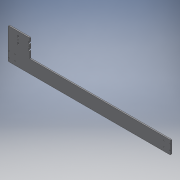
# Autodesk Inventor part: Wiper_Arm_1
Saved by Autodesk Inventor 2019 (Build 230136000, 136)
## iProperties
Created: 2020-03-11
Part Number: Wiper_Arm_1
Material: Generic
Document SubType Name: Modeling
Designer: Vijay
Density: 1 g/cm^3
Appearance: Default
Author: Vijay
Autodesk Inventor part; units mm, degrees
ref_plane "YZ Plane" through (0, 0, 0) normal (1, 0, 0) x (0, 1, 0)
ref_plane "XZ Plane" through (0, 0, 0) normal (0, 1, 0) x (-1, 0, 0)
ref_plane "XY Plane" through (0, 0, 0) normal (0, 0, 1) x (1, 0, 0)
sketch "Sketch1" plane through (0, 0, 0) normal (0, 0, 1) x (1, 0, 0)
  line L0 (19.3072, -32.4) -> (25.8072, -32.4) construction
  line L1 (25.8072, 0) -> (25.8072, -32.4) construction
  line L2 (19.3072, 0) -> (25.8072, 0) construction
  line L3 (19.3072, 0) -> (19.3072, -32.4) construction
  circle A0 centre (22.9072, -6.2) radius 1.75 construction
  circle A1 centre (22.9072, -26.2) radius 1.75 construction
  line L4 (0.0072, -32.4) -> (6.5072, -32.4) construction
  line L5 (6.5072, 0) -> (6.5072, -32.4) construction
  line L6 (0, 0) -> (6.5072, 0) construction
  line L7 (0.0072, 0) -> (0.0072, -32.4) projected
  circle A2 centre (2.9072, -6.2) radius 1.75 construction
  circle A3 centre (2.9072, -26.2) radius 1.75 construction
  line L8 (560.3075, -32.4001) -> (566.8075, -32.4001) construction
  line L9 (566.8075, -0.0001) -> (566.8075, -32.4001) projected
  line L10 (560.3075, -0.0001) -> (566.8075, -0.0001) construction
  line L11 (560.3075, -0.0001) -> (560.3075, -32.4001) construction
  circle A4 centre (563.9075, -6.2001) radius 1.75 construction
  circle A5 centre (563.9075, -26.2001) radius 1.75 construction
  line L12 (541.0075, -32.4001) -> (547.5075, -32.4001) construction
  line L13 (547.5075, -0.0001) -> (547.5075, -32.4001) construction
  line L14 (541.0075, -0.0001) -> (547.5075, -0.0001) construction
  line L15 (541.0075, -0.0001) -> (541.0075, -32.4001) construction
  circle A6 centre (543.9075, -6.2001) radius 1.75 construction
  circle A7 centre (543.9075, -26.2001) radius 1.75 construction
  line L16 (541.9075, 6.4999) -> (565.9075, 6.4999) projected
  line L17 (565.9075, -38.9001) -> (541.9075, -38.9001) projected
  line L18 (566.7649, -38.9) -> (0, -38.9)
  line L19 (0, -38.9) -> (0, 6.5)
  line L20 (0, 6.5) -> (566.7649, 6.5)
  line L21 (566.7649, 6.5) -> (566.7649, -38.9)
  circle A8 centre (563.9075, -26.2001) radius 1.5
  circle A9 centre (563.9075, -6.2001) radius 1.5
  circle A10 centre (543.9075, -26.2001) radius 1.5
  circle A11 centre (543.9075, -6.2001) radius 1.5
  circle A12 centre (22.9072, -26.2) radius 1.5
  circle A13 centre (22.9072, -6.2) radius 1.5
  circle A14 centre (2.9072, -26.2) radius 1.5
  circle A15 centre (2.9072, -6.2) radius 1.5
  point P0 (0, 0)
  dimension "d0" = 3
  dimension "d1" = 3
  dimension "d2" = 3
  dimension "d3" = 3
  dimension "d4" = 3
  dimension "d5" = 3
  dimension "d6" = 3
  dimension "d7" = 3
  constraints: 8 centre point, 8 coincident, 8 end point, 2 parallel, 1 horizontal, 1 perpendicular, 2 other
  measures "d0" diameter of A8
  measures "d1" diameter of A9
  measures "d2" diameter of A10
  measures "d3" diameter of A11
  measures "d4" diameter of A12
  measures "d5" diameter of A13
  measures "d6" diameter of A14
  measures "d7" diameter of A15
extrude "Extrusion1" add sketch "Sketch1" along normal blind 4
fillet "Fillet1" radius 2 4 edges at (566.7649, 6.5, 2) (566.7649, -38.9, 2) (0, -38.9, 2) (0, 6.5, 2)
sketch "Sketch2" plane through (0, 0, 4) normal (0, 0, 1) x (1, 0, 0)
  arc A0 (2, 6.5) -> (0, 4.5) centre (2, 4.5) ccw projected
  line L0 (0, 4.5) -> (0, -36.9) projected
  arc A1 (0, -36.9) -> (2, -38.9) centre (2, -36.9) ccw projected
  line L1 (2, -38.9) -> (564.7649, -38.9) projected
  arc A2 (564.7649, -38.9) -> (566.7649, -36.9) centre (564.7649, -36.9) ccw projected
  line L2 (566.7649, -36.9) -> (566.7649, 4.5) projected
  arc A3 (566.7649, 4.5) -> (564.7649, 6.5) centre (564.7649, 4.5) ccw projected
  line L3 (564.7649, 6.5) -> (2, 6.5) projected
  line L4 (0, 4.5) -> (0, -36.9) projected
  line L5 (0, 4.5) -> (74.776, 4.5)
  line L6 (74.776, 4.5) -> (74.776, 69.6091)
  line L7 (74.776, 69.6091) -> (0, 69.6091)
  line L8 (0, 69.6091) -> (0, 4.5)
  point P0 (0, 0)
  constraints: 8 end point, 2 parallel, 1 horizontal, 1 perpendicular
extrude "Extrusion2" add sketch "Sketch2" against normal up to surface (4 mm away) contours L3 L6 L5 A0 | A0 L8 L7 L6 L3
fillet "Fillet2" radius 2 2 edges at (0, 69.6091, 2) (74.776, 69.6091, 2)
fillet "Fillet3" radius 2 1 edges at (74.776, 6.5, 2)
sketch "Sketch3" plane through (0, 0, 0) normal (0, 0, -1) x (-1, 0, 0)
  line L0 (-32.9952, 56.8458) -> (-32.9952, 50.8458) construction
  line L1 (-32.9952, 56.8458) -> (-36.9952, 56.8458) construction
  line L2 (-36.9952, 50.8458) -> (-36.9952, 56.8458) construction
  line L3 (-32.9952, 50.8458) -> (-36.9952, 50.8458) construction
  line L4 (-32.9952, 35.6458) -> (-32.9952, 29.6458) construction
  line L5 (-32.9952, 35.6458) -> (-36.9952, 35.6458) construction
  line L6 (-36.9952, 29.6458) -> (-36.9952, 35.6458) construction
  line L7 (-32.9952, 29.6458) -> (-36.9952, 29.6458) construction
  line L8 (-70.776, 35.6458) -> (-70.776, 29.6458) construction
  line L9 (-70.776, 35.6458) -> (-74.776, 35.6458) construction
  line L10 (-74.776, 29.6458) -> (-74.776, 35.6458) construction
  line L11 (-70.776, 29.6458) -> (-74.776, 29.6458) construction
  line L12 (-70.776, 56.8458) -> (-70.776, 50.8458) construction
  line L13 (-70.776, 56.8458) -> (-74.776, 56.8458) construction
  line L14 (-74.776, 50.8458) -> (-74.776, 56.8458) construction
  line L15 (-70.776, 50.8458) -> (-74.776, 50.8458) construction
  line L16 (-36.9951, 41.5458) -> (-36.9951, 44.9458) construction
  line L17 (-32.9951, 41.5458) -> (-36.9951, 41.5458) construction
  line L18 (-32.9951, 44.9458) -> (-32.9951, 41.5458) construction
  line L19 (-32.9951, 44.9458) -> (-36.9951, 44.9458) construction
  line L20 (-74.776, 41.5458) -> (-74.776, 44.9458) construction
  line L21 (-70.776, 41.5458) -> (-74.776, 41.5458) construction
  line L22 (-70.776, 44.9458) -> (-70.776, 41.5458) construction
  line L23 (-70.776, 44.9458) -> (-74.776, 44.9458) construction
  line L24 (-74.976, 57.0458) -> (-70.576, 57.0458)
  line L25 (-70.576, 57.0458) -> (-70.576, 50.6458)
  line L26 (-70.576, 50.6458) -> (-74.976, 50.6458)
  line L27 (-74.976, 50.6458) -> (-74.976, 57.0458)
  line L28 (-74.976, 35.8458) -> (-70.576, 35.8458)
  line L29 (-70.576, 35.8458) -> (-70.576, 29.4458)
  line L30 (-70.576, 29.4458) -> (-74.976, 29.4458)
  line L31 (-74.976, 29.4458) -> (-74.976, 35.8458)
  line L32 (-37.1952, 57.0458) -> (-32.7952, 57.0458)
  line L33 (-32.7952, 57.0458) -> (-32.7952, 50.6458)
  line L34 (-32.7952, 50.6458) -> (-37.1952, 50.6458)
  line L35 (-37.1952, 50.6458) -> (-37.1952, 57.0458)
  line L36 (-37.1952, 35.8458) -> (-32.7952, 35.8458)
  line L37 (-32.7952, 35.8458) -> (-32.7952, 29.4458)
  line L38 (-32.7952, 29.4458) -> (-37.1952, 29.4458)
  line L39 (-37.1952, 29.4458) -> (-37.1952, 35.8458)
  circle A0 centre (-72.776, 43.2458) radius 1.6
  circle A1 centre (-34.988, 43.2458) radius 1.6
  point P0 (0, 0)
  dimension "d15" = 0.2
  dimension "d16" = 0.2
  dimension "d17" = 0.2
  dimension "d18" = 0.2
  dimension "d19" = 3.2
  dimension "d20" = 3.2
  constraints: 32 end point, 2 centre point, 12 other
  measures "d15" distance between parallel lines of L13 L24
  measures "d16" distance between parallel lines of L9 L28
  measures "d17" distance between parallel lines of L1 L32
  measures "d18" distance between parallel lines of L5 L36
  measures "d19" diameter of A0
  measures "d20" diameter of A1
extrude "Extrusion3" cut sketch "Sketch3" against normal blind 25.4
sketch "Sketch6" plane through (0, 0, 4) normal (0, 0, 1) x (1, 0, 0)
  line L0 (2, -38.9) -> (564.7649, -38.9) construction
  line L1 (282.6988, 626.8336) -> (282.6988, -296.2495) construction
  line L2 (497.6988, -38.9) -> (67.6988, -38.9)
  line L3 (67.6988, -38.9) -> (67.6988, -34.4)
  line L4 (67.6988, -34.4) -> (497.6988, -34.4)
  line L5 (497.6988, -34.4) -> (497.6988, -38.9)
  point P0 (0, 0)
  dimension "d29" = 4.5
  dimension "d30" = 430
  constraints: 10 end point, 2 parallel, 1 horizontal, 1 perpendicular, 1 point on line, 1 vertical, 1 other
  measures "d29" distance of L4.end L2.start
  measures "d30" distance of L3.end L4.end
extrude "Extrusion5" cut sketch "Sketch6" against normal blind 25.4
fillet "Fillet5" radius 1 2 edges at (497.6988, -38.9, 2) (67.6988, -38.9, 2)
sketch "Sketch7" plane through (0, 0, 4) normal (0, 0, 1) x (1, 0, 0)
  arc A0 (214.4105, 1.0634) -> (213.9105, 1.5634) centre (213.9105, 1.0634) ccw construction
  line L0 (213.9105, 1.5634) -> (210.4105, 1.5634) construction
  line L1 (210.4105, 1.5634) -> (210.4105, 8.4392) construction
  line L2 (210.4105, 8.4392) -> (201.1321, 8.4392) construction
  arc A1 (201.1321, 8.4392) -> (199.8552, 7.9785) centre (201.1321, 6.4392) ccw construction
  line L3 (199.8552, 7.9785) -> (161.5461, -23.8002) construction
  arc A2 (161.5461, -23.8002) -> (160.823, -25.3395) centre (162.823, -25.3395) ccw construction
  line L4 (160.823, -25.3395) -> (160.823, -34.4) projected
  line L5 (160.823, -34.4) -> (167.6988, -34.4) projected
  line L6 (167.6988, -34.4) -> (167.6988, -37.9) projected
  arc A3 (167.6988, -37.9) -> (168.1988, -38.4) centre (168.1988, -37.9) ccw projected
  line L7 (168.1988, -38.4) -> (173.1988, -38.4) projected
  arc A4 (173.1988, -38.4) -> (173.6988, -37.9) centre (173.1988, -37.9) ccw projected
  line L8 (173.6988, -37.9) -> (173.6988, -34.4) projected
  line L9 (173.6988, -34.4) -> (179.5988, -34.4) projected
  line L10 (179.5988, -34.4) -> (179.5988, -28.6) projected
  line L11 (179.5988, -28.6) -> (178.3488, -28.6) construction
  line L12 (178.3488, -28.6) -> (178.3488, -26.2) construction
  line L13 (178.3488, -26.2) -> (179.5988, -26.2) construction
  line L14 (179.5988, -26.2) -> (179.5988, -23.55) construction
  line L15 (179.5988, -23.55) -> (182.9988, -23.55) construction
  line L16 (182.9988, -23.55) -> (182.9988, -26.2) construction
  line L17 (182.9988, -26.2) -> (184.2488, -26.2) construction
  line L18 (184.2488, -26.2) -> (184.2488, -28.6) construction
  line L19 (184.2488, -28.6) -> (182.9988, -28.6) construction
  line L20 (182.9988, -28.6) -> (182.9988, -34.4) projected
  line L21 (182.9988, -34.4) -> (188.8988, -34.4) projected
  line L22 (188.8988, -34.4) -> (188.8988, -37.9) projected
  arc A5 (188.8988, -37.9) -> (189.3988, -38.4) centre (189.3988, -37.9) ccw projected
  line L23 (189.3988, -38.4) -> (194.3988, -38.4) projected
  arc A6 (194.3988, -38.4) -> (194.8988, -37.9) centre (194.3988, -37.9) ccw projected
  line L24 (194.8988, -37.9) -> (194.8988, -34.4) projected
  line L25 (194.8988, -34.4) -> (210.4105, -34.4) projected
  line L26 (210.4105, -34.4) -> (210.4105, -25.6366) projected
  line L27 (210.4105, -25.6366) -> (213.9105, -25.6366) construction
  arc A7 (213.9105, -25.6366) -> (214.4105, -25.1366) centre (213.9105, -25.1366) ccw construction
  line L28 (214.4105, -25.1366) -> (214.4105, -20.1366) construction
  arc A8 (214.4105, -20.1366) -> (213.9105, -19.6366) centre (213.9105, -20.1366) ccw construction
  line L29 (213.9105, -19.6366) -> (210.4105, -19.6366) construction
  line L30 (210.4105, -19.6366) -> (210.4105, -13.7366) construction
  line L31 (210.4105, -13.7366) -> (204.6105, -13.7366) construction
  line L32 (204.6105, -13.7366) -> (204.6105, -14.9866) construction
  line L33 (204.6105, -14.9866) -> (202.2105, -14.9866) construction
  line L34 (202.2105, -14.9866) -> (202.2105, -13.7366) construction
  line L35 (202.2105, -13.7366) -> (199.5605, -13.7366) construction
  line L36 (199.5605, -13.7366) -> (199.5605, -10.3366) construction
  line L37 (199.5605, -10.3366) -> (202.2105, -10.3366) construction
  line L38 (202.2105, -10.3366) -> (202.2105, -9.0866) construction
  line L39 (202.2105, -9.0866) -> (204.6105, -9.0866) construction
  line L40 (204.6105, -9.0866) -> (204.6105, -10.3366) construction
  line L41 (204.6105, -10.3366) -> (210.4105, -10.3366) construction
  line L42 (210.4105, -10.3366) -> (210.4105, -4.4366) construction
  line L43 (210.4105, -4.4366) -> (213.9105, -4.4366) construction
  arc A9 (213.9105, -4.4366) -> (214.4105, -3.9366) centre (213.9105, -3.9366) ccw construction
  line L44 (214.4105, -3.9366) -> (214.4105, 1.0634) construction
  arc A10 (417.2105, 1.0634) -> (416.7105, 1.5634) centre (416.7105, 1.0634) ccw construction
  line L45 (416.7105, 1.5634) -> (413.2105, 1.5634) construction
  line L46 (413.2105, 1.5634) -> (413.2105, 8.4392) construction
  line L47 (413.2105, 8.4392) -> (403.9321, 8.4392) construction
  arc A11 (403.9321, 8.4392) -> (402.6552, 7.9785) centre (403.9321, 6.4392) ccw construction
  line L48 (402.6552, 7.9785) -> (364.3461, -23.8002) construction
  arc A12 (364.3461, -23.8002) -> (363.623, -25.3395) centre (365.623, -25.3395) ccw construction
  line L49 (363.623, -25.3395) -> (363.623, -34.4) projected
  line L50 (363.623, -34.4) -> (370.4988, -34.4) projected
  line L51 (370.4988, -34.4) -> (370.4988, -37.9) projected
  arc A13 (370.4988, -37.9) -> (370.9988, -38.4) centre (370.9988, -37.9) ccw projected
  line L52 (370.9988, -38.4) -> (375.9988, -38.4) projected
  arc A14 (375.9988, -38.4) -> (376.4988, -37.9) centre (375.9988, -37.9) ccw projected
  line L53 (376.4988, -37.9) -> (376.4988, -34.4) projected
  line L54 (376.4988, -34.4) -> (382.3988, -34.4) projected
  line L55 (382.3988, -34.4) -> (382.3988, -28.6) projected
  line L56 (382.3988, -28.6) -> (381.1488, -28.6) construction
  line L57 (381.1488, -28.6) -> (381.1488, -26.2) construction
  line L58 (381.1488, -26.2) -> (382.3988, -26.2) construction
  line L59 (382.3988, -26.2) -> (382.3988, -23.55) construction
  line L60 (382.3988, -23.55) -> (385.7988, -23.55) construction
  line L61 (385.7988, -23.55) -> (385.7988, -26.2) construction
  line L62 (385.7988, -26.2) -> (387.0488, -26.2) construction
  line L63 (387.0488, -26.2) -> (387.0488, -28.6) construction
  line L64 (387.0488, -28.6) -> (385.7988, -28.6) construction
  line L65 (385.7988, -28.6) -> (385.7988, -34.4) projected
  line L66 (385.7988, -34.4) -> (391.6988, -34.4) projected
  line L67 (391.6988, -34.4) -> (391.6988, -37.9) projected
  arc A15 (391.6988, -37.9) -> (392.1988, -38.4) centre (392.1988, -37.9) ccw projected
  line L68 (392.1988, -38.4) -> (397.1988, -38.4) projected
  arc A16 (397.1988, -38.4) -> (397.6988, -37.9) centre (397.1988, -37.9) ccw projected
  line L69 (397.6988, -37.9) -> (397.6988, -34.4) projected
  line L70 (397.6988, -34.4) -> (413.2105, -34.4) projected
  line L71 (413.2105, -34.4) -> (413.2105, -25.6366) projected
  line L72 (413.2105, -25.6366) -> (416.7105, -25.6366) construction
  arc A17 (416.7105, -25.6366) -> (417.2105, -25.1366) centre (416.7105, -25.1366) ccw construction
  line L73 (417.2105, -25.1366) -> (417.2105, -20.1366) construction
  arc A18 (417.2105, -20.1366) -> (416.7105, -19.6366) centre (416.7105, -20.1366) ccw construction
  line L74 (416.7105, -19.6366) -> (413.2105, -19.6366) construction
  line L75 (413.2105, -19.6366) -> (413.2105, -13.7366) construction
  line L76 (413.2105, -13.7366) -> (407.4105, -13.7366) construction
  line L77 (407.4105, -13.7366) -> (407.4105, -14.9866) construction
  line L78 (407.4105, -14.9866) -> (405.0105, -14.9866) construction
  line L79 (405.0105, -14.9866) -> (405.0105, -13.7366) construction
  line L80 (405.0105, -13.7366) -> (402.3605, -13.7366) construction
  line L81 (402.3605, -13.7366) -> (402.3605, -10.3366) construction
  line L82 (402.3605, -10.3366) -> (405.0105, -10.3366) construction
  line L83 (405.0105, -10.3366) -> (405.0105, -9.0866) construction
  line L84 (405.0105, -9.0866) -> (407.4105, -9.0866) construction
  line L85 (407.4105, -9.0866) -> (407.4105, -10.3366) construction
  line L86 (407.4105, -10.3366) -> (413.2105, -10.3366) construction
  line L87 (413.2105, -10.3366) -> (413.2105, -4.4366) construction
  line L88 (413.2105, -4.4366) -> (416.7105, -4.4366) construction
  arc A19 (416.7105, -4.4366) -> (417.2105, -3.9366) centre (416.7105, -3.9366) ccw construction
  line L89 (417.2105, -3.9366) -> (417.2105, 1.0634) construction
  line L90 (67.6988, -34.4) -> (497.6988, -34.4) projected
  line L91 (167.6988, -34.4) -> (173.6988, -34.4)
  line L92 (179.5988, -34.4) -> (182.9988, -34.4)
  line L93 (188.8988, -34.4) -> (194.8988, -34.4)
  line L94 (391.6988, -34.4) -> (397.6988, -34.4)
  line L95 (382.3988, -34.4) -> (385.7988, -34.4)
  line L96 (210.4105, -34.4) -> (363.623, -34.4)
  line L97 (370.4988, -34.4) -> (376.4988, -34.4)
  point P0 (0, 0)
  constraints: 26 end point, 7 horizontal, 2 point on line, 1 other
extrude "Extrusion6" add sketch "Sketch7" against normal up to surface (4 mm away)
sketch "Sketch8" plane through (0, 0, 4) normal (0, 0, 1) x (1, 0, 0)
  arc A0 (214.4105, 1.0634) -> (213.9105, 1.5634) centre (213.9105, 1.0634) ccw construction
  line L0 (213.9105, 1.5634) -> (210.4105, 1.5634) construction
  line L1 (210.4105, 1.5634) -> (210.4105, 8.4392) construction
  line L2 (210.4105, 8.4392) -> (201.1321, 8.4392) construction
  arc A1 (201.1321, 8.4392) -> (199.8552, 7.9785) centre (201.1321, 6.4392) ccw construction
  line L3 (199.8552, 7.9785) -> (161.5461, -23.8002) projected
  arc A2 (161.5461, -23.8002) -> (160.823, -25.3395) centre (162.823, -25.3395) ccw construction
  line L4 (160.823, -25.3395) -> (160.823, -34.4) construction
  line L5 (160.823, -34.4) -> (167.6988, -34.4) construction
  line L6 (167.6988, -34.4) -> (167.6988, -37.9) construction
  arc A3 (167.6988, -37.9) -> (168.1988, -38.4) centre (168.1988, -37.9) ccw construction
  line L7 (168.1988, -38.4) -> (173.1988, -38.4) construction
  arc A4 (173.1988, -38.4) -> (173.6988, -37.9) centre (173.1988, -37.9) ccw construction
  line L8 (173.6988, -37.9) -> (173.6988, -34.4) construction
  line L9 (173.6988, -34.4) -> (179.5988, -34.4) projected
  line L10 (179.5988, -34.4) -> (179.5988, -28.6) projected
  line L11 (179.5988, -28.6) -> (178.3488, -28.6) projected
  line L12 (178.3488, -28.6) -> (178.3488, -26.2) projected
  line L13 (178.3488, -26.2) -> (179.5988, -26.2) projected
  line L14 (179.5988, -26.2) -> (179.5988, -23.55) projected
  line L15 (179.5988, -23.55) -> (182.9988, -23.55) projected
  line L16 (182.9988, -23.55) -> (182.9988, -26.2) projected
  line L17 (182.9988, -26.2) -> (184.2488, -26.2) projected
  line L18 (184.2488, -26.2) -> (184.2488, -28.6) projected
  line L19 (184.2488, -28.6) -> (182.9988, -28.6) projected
  line L20 (182.9988, -28.6) -> (182.9988, -34.4) projected
  line L21 (182.9988, -34.4) -> (188.8988, -34.4) projected
  line L22 (188.8988, -34.4) -> (188.8988, -37.9) projected
  arc A5 (188.8988, -37.9) -> (189.3988, -38.4) centre (189.3988, -37.9) ccw projected
  line L23 (189.3988, -38.4) -> (194.3988, -38.4) projected
  arc A6 (194.3988, -38.4) -> (194.8988, -37.9) centre (194.3988, -37.9) ccw projected
  line L24 (194.8988, -37.9) -> (194.8988, -34.4) projected
  line L25 (194.8988, -34.4) -> (210.4105, -34.4) projected
  line L26 (210.4105, -34.4) -> (210.4105, -25.6366) projected
  line L27 (210.4105, -25.6366) -> (213.9105, -25.6366) projected
  arc A7 (213.9105, -25.6366) -> (214.4105, -25.1366) centre (213.9105, -25.1366) ccw projected
  line L28 (214.4105, -25.1366) -> (214.4105, -20.1366) projected
  arc A8 (214.4105, -20.1366) -> (213.9105, -19.6366) centre (213.9105, -20.1366) ccw construction
  line L29 (213.9105, -19.6366) -> (210.4105, -19.6366) construction
  line L30 (210.4105, -19.6366) -> (210.4105, -13.7366) construction
  line L31 (210.4105, -13.7366) -> (204.6105, -13.7366) construction
  line L32 (204.6105, -13.7366) -> (204.6105, -14.9866) construction
  line L33 (204.6105, -14.9866) -> (202.2105, -14.9866) construction
  line L34 (202.2105, -14.9866) -> (202.2105, -13.7366) construction
  line L35 (202.2105, -13.7366) -> (199.5605, -13.7366) construction
  line L36 (199.5605, -13.7366) -> (199.5605, -10.3366) construction
  line L37 (199.5605, -10.3366) -> (202.2105, -10.3366) construction
  line L38 (202.2105, -10.3366) -> (202.2105, -9.0866) construction
  line L39 (202.2105, -9.0866) -> (204.6105, -9.0866) construction
  line L40 (204.6105, -9.0866) -> (204.6105, -10.3366) construction
  line L41 (204.6105, -10.3366) -> (210.4105, -10.3366) construction
  line L42 (210.4105, -10.3366) -> (210.4105, -4.4366) construction
  line L43 (210.4105, -4.4366) -> (213.9105, -4.4366) construction
  arc A9 (213.9105, -4.4366) -> (214.4105, -3.9366) centre (213.9105, -3.9366) ccw construction
  line L44 (214.4105, -3.9366) -> (214.4105, 1.0634) construction
  arc A10 (417.2105, 1.0634) -> (416.7105, 1.5634) centre (416.7105, 1.0634) ccw construction
  line L45 (416.7105, 1.5634) -> (413.2105, 1.5634) construction
  line L46 (413.2105, 1.5634) -> (413.2105, 8.4392) construction
  line L47 (413.2105, 8.4392) -> (403.9321, 8.4392) construction
  arc A11 (403.9321, 8.4392) -> (402.6552, 7.9785) centre (403.9321, 6.4392) ccw construction
  line L48 (402.6552, 7.9785) -> (364.3461, -23.8002) construction
  arc A12 (364.3461, -23.8002) -> (363.623, -25.3395) centre (365.623, -25.3395) ccw construction
  line L49 (363.623, -25.3395) -> (363.623, -34.4) construction
  line L50 (363.623, -34.4) -> (370.4988, -34.4) construction
  line L51 (370.4988, -34.4) -> (370.4988, -37.9) construction
  arc A13 (370.4988, -37.9) -> (370.9988, -38.4) centre (370.9988, -37.9) ccw construction
  line L52 (370.9988, -38.4) -> (375.9988, -38.4) construction
  arc A14 (375.9988, -38.4) -> (376.4988, -37.9) centre (375.9988, -37.9) ccw construction
  line L53 (376.4988, -37.9) -> (376.4988, -34.4) construction
  line L54 (376.4988, -34.4) -> (382.3988, -34.4) projected
  line L55 (382.3988, -34.4) -> (382.3988, -28.6) projected
  line L56 (382.3988, -28.6) -> (381.1488, -28.6) projected
  line L57 (381.1488, -28.6) -> (381.1488, -26.2) projected
  line L58 (381.1488, -26.2) -> (382.3988, -26.2) projected
  line L59 (382.3988, -26.2) -> (382.3988, -23.55) projected
  line L60 (382.3988, -23.55) -> (385.7988, -23.55) projected
  line L61 (385.7988, -23.55) -> (385.7988, -26.2) projected
  line L62 (385.7988, -26.2) -> (387.0488, -26.2) projected
  line L63 (387.0488, -26.2) -> (387.0488, -28.6) projected
  line L64 (387.0488, -28.6) -> (385.7988, -28.6) projected
  line L65 (385.7988, -28.6) -> (385.7988, -34.4) projected
  line L66 (385.7988, -34.4) -> (391.6988, -34.4) projected
  line L67 (391.6988, -34.4) -> (391.6988, -37.9) projected
  arc A15 (391.6988, -37.9) -> (392.1988, -38.4) centre (392.1988, -37.9) ccw construction
  line L68 (392.1988, -38.4) -> (397.1988, -38.4) construction
  arc A16 (397.1988, -38.4) -> (397.6988, -37.9) centre (397.1988, -37.9) ccw construction
  line L69 (397.6988, -37.9) -> (397.6988, -34.4) construction
  line L70 (397.6988, -34.4) -> (413.2105, -34.4) construction
  line L71 (413.2105, -34.4) -> (413.2105, -25.6366) construction
  line L72 (413.2105, -25.6366) -> (416.7105, -25.6366) construction
  arc A17 (416.7105, -25.6366) -> (417.2105, -25.1366) centre (416.7105, -25.1366) ccw construction
  line L73 (417.2105, -25.1366) -> (417.2105, -20.1366) construction
  arc A18 (417.2105, -20.1366) -> (416.7105, -19.6366) centre (416.7105, -20.1366) ccw construction
  line L74 (416.7105, -19.6366) -> (413.2105, -19.6366) construction
  line L75 (413.2105, -19.6366) -> (413.2105, -13.7366) construction
  line L76 (413.2105, -13.7366) -> (407.4105, -13.7366) construction
  line L77 (407.4105, -13.7366) -> (407.4105, -14.9866) construction
  line L78 (407.4105, -14.9866) -> (405.0105, -14.9866) construction
  line L79 (405.0105, -14.9866) -> (405.0105, -13.7366) construction
  line L80 (405.0105, -13.7366) -> (402.3605, -13.7366) construction
  line L81 (402.3605, -13.7366) -> (402.3605, -10.3366) construction
  line L82 (402.3605, -10.3366) -> (405.0105, -10.3366) construction
  line L83 (405.0105, -10.3366) -> (405.0105, -9.0866) construction
  line L84 (405.0105, -9.0866) -> (407.4105, -9.0866) construction
  line L85 (407.4105, -9.0866) -> (407.4105, -10.3366) construction
  line L86 (407.4105, -10.3366) -> (413.2105, -10.3366) construction
  line L87 (413.2105, -10.3366) -> (413.2105, -4.4366) construction
  line L88 (413.2105, -4.4366) -> (416.7105, -4.4366) construction
  arc A19 (416.7105, -4.4366) -> (417.2105, -3.9366) centre (416.7105, -3.9366) ccw construction
  line L89 (417.2105, -3.9366) -> (417.2105, 1.0634) construction
  line L90 (179.5988, -34.4) -> (182.9988, -34.4)
  line L91 (188.8988, -34.4) -> (173.6988, -34.4) projected
  line L92 (382.3988, -34.4) -> (385.7988, -34.4)
  line L93 (391.6988, -34.4) -> (376.4988, -34.4) projected
  point P0 (0, 0)
  constraints: 4 end point, 2 collinear
extrude "Extrusion7" cut sketch "Sketch8" against normal blind 25.4
body "Solid1"
